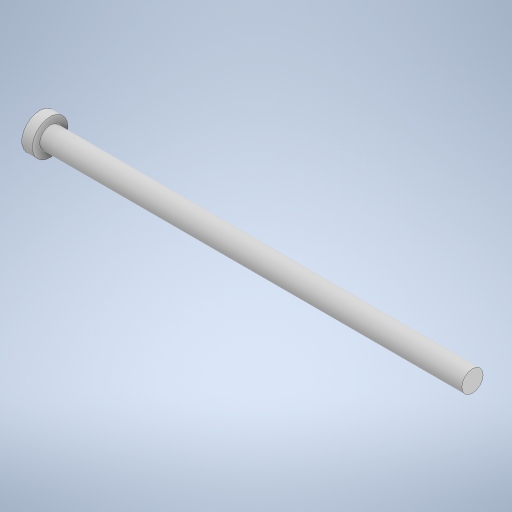
# Autodesk Inventor part: Part7
Saved by Autodesk Inventor 2024 (Build 280153000, 153)
## iProperties
Created: 2023-12-18
Part Number: Part7
Material: Generic
Document SubType Name: Modeling
Designer: SAHITYA
Density: 1 g/cm^3
Appearance: Default
Author: SAHITYA
Autodesk Inventor part; units mm, degrees
ref_plane "YZ Plane" through (0, 0, 0) normal (1, 0, 0) x (0, 1, 0)
ref_plane "XZ Plane" through (0, 0, 0) normal (0, 1, 0) x (-1, 0, 0)
ref_plane "XY Plane" through (0, 0, 0) normal (0, 0, 1) x (1, 0, 0)
sketch "Sketch1" plane through (0, 0, 0) normal (0, 1, 0) x (-1, 0, 0)
  line L0 (16.9868, 0.0221) -> (-8.0132, 0.0221)
  line L1 (-8.0132, 0.0221) -> (-8.0132, -1.4779)
  line L2 (-8.0132, -1.4779) -> (16.9868, -1.4779)
  line L3 (16.9868, -1.4779) -> (16.9868, 0.0221)
  line L4 (16.9868, 0.0221) -> (16.9868, -2.4779)
  line L5 (16.9868, -2.4779) -> (18.4868, -2.4779)
  line L6 (18.4868, -2.4779) -> (18.4868, 0.0221)
  line L7 (18.4868, 0.0221) -> (16.9868, 0.0221)
  line L8 (16.9868, 0.0221) -> (-30.5132, 0.0221)
  line L9 (-30.5132, 0.0221) -> (-35.5132, 0.0221)
  line L10 (-35.5132, 0.0221) -> (-35.5132, -1.4779)
  line L11 (-35.5132, -1.4779) -> (-8.0132, -1.4779)
  line L12 (-35.5132, 0.0221) -> (-40.5132, 0.0221)
  line L13 (-40.5132, 0.0221) -> (-40.5132, -1.4779)
  line L14 (-40.5132, -1.4779) -> (-35.5132, -1.4779)
  line L15 (-40.5132, 0.0221) -> (-42.5134, 0.0221)
  line L16 (-42.5134, 0.0221) -> (-42.5134, -1.4779)
  line L17 (-42.5134, -1.4779) -> (-40.5132, -1.4779)
  dimension "d3" = 25
  dimension "d4" = 1.5
  dimension "d5" = 2.5
  dimension "d6" = 1.5
  dimension "d7" = 47.5
  dimension "d8" = 5
  dimension "d10" = 5
  constraints: 36 end point, 12 perpendicular, 4 point on line, 3 horizontal
  measures "d3" distance of L0.start L0.end
  measures "d4" distance of L0.end L1.end
  measures "d5" distance of L0.start L4.end
  measures "d6" distance of L4.end L5.end
  measures "d7" distance of L0.start L8.end
  measures "d8" distance of L8.end L9.end
  measures "d10" distance of L9.end L12.end
revolve "Revolution1" add sketch "Sketch1" angle 360 about axis through (-16.9868, 0, 0.0221) along (1, 0, 0)
body "Solid1"
